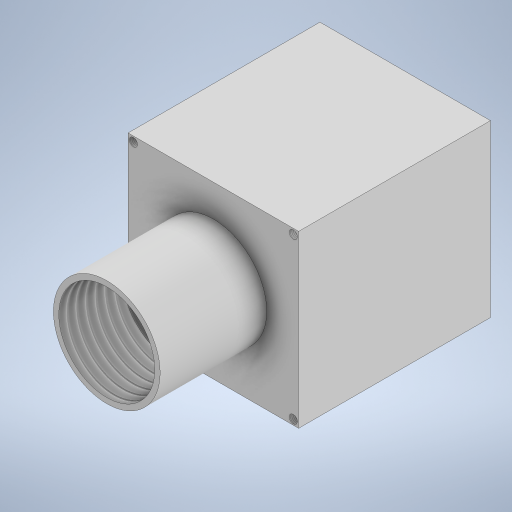
# Autodesk Inventor part: PRACTICA 1
Saved by Autodesk Inventor 2024 (Build 280153000, 153)
## iProperties
Created: 2024-01-23
Part Number: PRACTICA 1
Material: Genérico
Document SubType Name: Modeling
Designer: Adrian Montalvan
Density: 1 g/cm^3
Appearance: Valor por defecto
Author: Adrian Montalvan
Autodesk Inventor part; units mm, degrees
ref_plane "YZ Plane" through (0, 0, 0) normal (1, 0, 0) x (0, 1, 0)
ref_plane "XZ Plane" through (0, 0, 0) normal (0, 1, 0) x (-1, 0, 0)
ref_plane "XY Plane" through (0, 0, 0) normal (0, 0, 1) x (1, 0, 0)
sketch "Boceto1" plane through (0, 0, 0) normal (0, 0, 1) x (1, 0, 0)
  line L0 (-40, -40) -> (40, -40)
  line L1 (40, -40) -> (40, 40)
  line L2 (40, 40) -> (-40, 40)
  line L3 (-40, 40) -> (-40, -40)
  line L4 (-40, -40) -> (40, 40) construction
  line L5 (40, -40) -> (-40, 40) construction
  point P0 (0, 0)
  dimension "d0" = 80
  dimension "d1" = 80
  constraints: 12 end point, 2 midpoint, 2 parallel, 1 horizontal, 1 perpendicular
  measures "d0" distance of L2.end L1.end
  measures "d1" distance of L1.end L0.end
extrude "Extrusión1" add sketch "Boceto1" along normal blind 90
sketch "Boceto2" plane through (0, 0, 90) normal (0, 0, 1) x (1, 0, 0)
  circle A0 centre (0, 0) radius 25
  circle A1 centre (0, 0) radius 22.5
  dimension "d4" = 50
  dimension "d5" = 45
  constraints: 2 centre point, 2 coincident
  measures "d4" diameter of A0
  measures "d5" diameter of A1
extrude "Extrusión2" add sketch "Boceto2" along normal blind 50
sketch "Boceto3" plane through (0, 0, 0) normal (0, 0, -1) x (-1, 0, 0)
  line L0 (-35, -35) -> (35, -35)
  line L1 (35, -35) -> (35, 35)
  line L2 (35, 35) -> (-35, 35)
  line L3 (-35, 35) -> (-35, -35)
  line L4 (-35, -35) -> (35, 35) construction
  line L5 (35, -35) -> (-35, 35) construction
  line L6 (-40, 40) -> (40, 40) projected
  line L7 (-40, -40) -> (-40, 40) projected
  circle A0 centre (-37.5, 37.5) radius 1.9
  circle A1 centre (37.5, 37.5) radius 1.9
  circle A2 centre (37.5, -37.5) radius 1.9
  circle A3 centre (-37.5, -37.5) radius 1.9
  point P0 (0, 0)
  dimension "d9" = 70
  constraints: 12 end point, 4 centre point, 2 midpoint, 2 parallel, 1 horizontal, 1 perpendicular
  measures "d9" distance of L1.end L0.end
sketch "Boceto4" plane through (0, 0, 0) normal (0, 0, -1) x (-1, 0, 0)
  point P0 (0, 0)
extrude "Extrusión3" cut sketch "Boceto3" against normal blind 90 contours A0 | A1 | A2 | A3
sketch "Boceto5" plane through (0, 0, 90) normal (0, 0, 1) x (1, 0, 0)
  circle A0 centre (0, 0) radius 22.5
  dimension "d14" = 45
  constraints: 1 centre point, 1 coincident
  measures "d14" diameter of A0
extrude "Extrusión4" add sketch "Boceto5" along normal blind 20
thread "Rosca1" size "M4x0.7" class "6H" standard "ANSI Metric M Profile" full length
thread "Rosca2" size "M4x0.7" class "6H" standard "ANSI Metric M Profile" full length
thread "Rosca3" size "M4x0.7" class "6H" standard "ANSI Metric M Profile" full length
thread "Rosca4" size "M4x0.7" class "6H" standard "ANSI Metric M Profile" full length
thread "Rosca5" size "M45x4.5" class "6H" standard "ANSI Metric M Profile" full length
